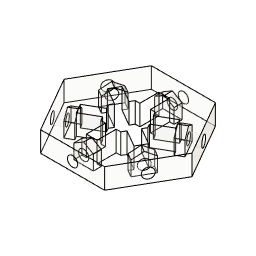
CapacitorJig (Autodesk Fusion 360 design; units mm, degrees)
Autodesk Fusion 360 part; units mm, degrees
note: some values were not read from the file. Chosen so that the rebuilt part matches the saved one: a direction; which face or edge a step refers to. Set by a fixed rule: which sketch regions a step uses.
sketch "Sketch1" plane through (0, 0, 0) normal (0, 0, 1) x (1, 0, 0)
  line L0 (-5.4993, 9.525) -> (-10.9985, 0)
  line L1 (-10.9985, 0) -> (-5.4993, -9.525)
  line L2 (-5.4993, -9.525) -> (5.4993, -9.525)
  line L3 (5.4993, -9.525) -> (10.9985, 0)
  line L4 (10.9985, 0) -> (5.4993, 9.525)
  line L5 (5.4993, 9.525) -> (-5.4993, 9.525)
  line L6 (-8.386, -14.525) -> (8.386, -14.525)
  line L7 (8.386, -14.525) -> (16.772, 0)
  line L8 (16.772, 0) -> (8.386, 14.525)
  line L9 (8.386, 14.525) -> (-8.386, 14.525)
  line L10 (-8.386, 14.525) -> (-16.772, 0)
  line L11 (-16.772, 0) -> (-8.386, -14.525)
  dimension "d1" = 19.05
  dimension "d2" = 5
  measures "d1" distance of L2 L5
extrude "Extrude1" add sketch "Sketch1" along normal blind 5.35
sketch "Sketch2" plane through (0, 0, 5.35) normal (0, 0, 1) x (-1, 0, 0)
  line L0 (5.4993, -9.525) -> (-5.4993, -9.525)
  line L1 (-5.4993, -9.525) -> (-10.9985, 0)
  line L2 (-10.9985, 0) -> (-5.4993, 9.525)
  line L3 (-5.4993, 9.525) -> (5.4993, 9.525)
  line L4 (5.4993, 9.525) -> (10.9985, 0)
  line L5 (10.9985, 0) -> (5.4993, -9.525)
  line L6 (16.772, 0) -> (8.386, 14.525)
  line L7 (8.386, 14.525) -> (-8.386, 14.525)
  line L8 (-8.386, 14.525) -> (-16.772, 0)
  line L9 (-16.772, 0) -> (-8.386, -14.525)
  line L10 (-8.386, -14.525) -> (8.386, -14.525)
  line L11 (8.386, -14.525) -> (16.772, 0)
  line L12 (1.4, -9.525) -> (1.4, -2.4249)
  line L13 (1.4, -2.4249) -> (7.5489, -5.9749)
  dimension "d5" = 1.4
  constraint perpendicular L10 L12
  constraint coincident L0 L12.start
  constraint coincident L5 L13.end
  constraint perpendicular L5 L13
  constraint equal L12 L13
  measures "d5" horizontal distance of origin L12.start
extrude "Extrude2" add sketch "Sketch2" against normal up to surface (5.35 mm away) contours L0 L5 L12 L13
pattern_circular "C-Pattern1" count 6 over 360 about axis through (0, 0, 1.75) along (0, 0, 1) of "Extrude2"
sketch "Sketch3" plane through (0, 14.525, 0) normal (0, 1, 0) x (-1, 0, 0)
  line L0 (-8.386, 0) -> (8.386, 0)
  line L1 (8.386, 0) -> (8.386, 5.35)
  line L2 (8.386, 5.35) -> (-8.386, 5.35)
  line L3 (-8.386, 5.35) -> (-8.386, 0)
  point P0 (0, 2.35)
  point P1 (8.386, 2.675)
  dimension "d21" = 3
  constraint midpoint L1 P1
  measures "d21" distance of L2 P0
hole "Hole1" at (0, 14.525, 2.35) direction (0, -1, 0) diameter 2.7 end through all
pattern_circular "C-Pattern2" count 3 over 360 about axis through (0, 0, 1.75) along (0, 0, 1) of "Hole1"
sketch "Sketch4" plane through (8.2489, -4.7625, 0) normal (-0.866025, 0.5, 0) x (-0.5, -0.866025, 0)
  line L0 (-1.4, 5.35) -> (-1.4, 0)
  line L1 (-1.4, 0) -> (1.4, 0)
  line L2 (1.4, 0) -> (1.4, 5.35)
  line L3 (1.4, 5.35) -> (-1.4, 5.35)
  line L4 (-2.55, 0.8778) -> (0, -0.5945)
  line L5 (0, -0.5945) -> (2.55, 0.8778)
  line L6 (2.55, 0.8778) -> (2.55, 3.8222)
  line L7 (2.55, 3.8222) -> (0, 5.2945)
  line L8 (0, 5.2945) -> (-2.55, 3.8222)
  line L9 (-2.55, 3.8222) -> (-2.55, 0.8778)
  line L10 (-2.55, 0.8778) -> (-2.55, -0.825)
  line L11 (-2.55, -0.825) -> (2.55, -0.825)
  line L12 (2.55, -0.825) -> (2.55, 0.8778)
  circle A0 centre (0, 2.35) radius 1.35
  point P0 (0, 2.35)
  dimension "d15" = 5.1
  constraint coincident P0 A0.centre
  constraint vertical L9
  constraint parallel L9 L10
  constraint perpendicular L0 L11
  constraint vertical L12
  measures "d15" distance of L6 L9
extrude "Extrude3" cut sketch "Sketch4" against normal blind 2.1 contours L0 L1 L2 L4 L5 L7 L8 | L0 L4 L8 L9 | L0 L1 L4 | L0 L1 L2 L4 L5 L10 L11 L12 | L2 L5 L6 L7 | L1 L4 L5 | L1 L2 L5
pattern_circular "C-Pattern3" count 6 over 360 about axis through (0, 0, 1.75) along (0, 0, 1) of "Extrude3"
sketch "Sketch5" plane through (0, 0, 0) normal (0, 0, 1) x (1, 0, 0)
  line L0 (2.5981, -4.5) -> (5.1962, 0)
  line L1 (5.1962, 0) -> (2.5981, 4.5)
  line L2 (2.5981, 4.5) -> (-2.5981, 4.5)
  line L3 (-2.5981, 4.5) -> (-5.1962, 0)
  line L4 (-5.1962, 0) -> (-2.5981, -4.5)
  line L5 (-2.5981, -4.5) -> (2.5981, -4.5)
  dimension "d22" = 9
  constraint horizontal L5
  measures "d22" distance of L2 L5
extrude "Extrude4" cut sketch "Sketch5" along normal through all
